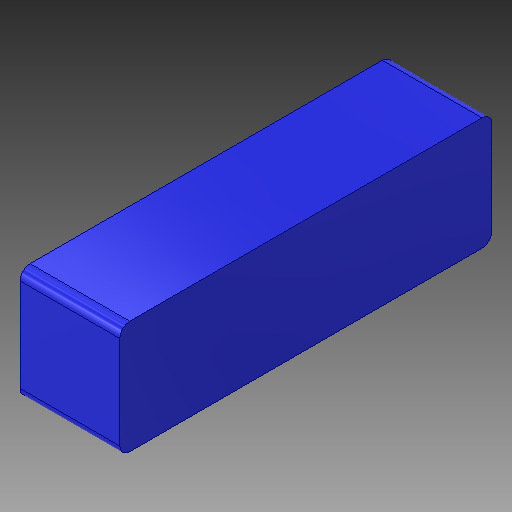
# Autodesk Inventor part: battery
Saved by Autodesk Inventor 2018 (Build 220112000, 112)
## iProperties
Created: 2016-04-08
Part Number: battery
Material: Generic
Document SubType Name: Modeling
Designer: steve
Density: 2.20668 g/cm^3
Appearance: Blue - Wall Paint - Glossy
Mass: 220 g
Surface Area: 147.334 cm^2
Volume: 99.6973 cm^3
Vendor: HobbyKing
Provider: HobbyKing
Author: steve
Autodesk Inventor part; units mm, degrees
ref_plane "YZ Plane" through (0, 0, 0) normal (1, 0, 0) x (0, 1, 0)
ref_plane "XZ Plane" through (0, 0, 0) normal (0, 1, 0) x (-1, 0, 0)
ref_plane "XY Plane" through (0, 0, 0) normal (0, 0, 1) x (1, 0, 0)
sketch "Sketch1" plane through (0, 0, 0) normal (0, 1, 0) x (-1, 0, 0)
  line L0 (-15, 56) -> (15, 56)
  line L1 (15, 56) -> (15, -56)
  line L2 (15, -56) -> (-15, -56)
  line L3 (-15, -56) -> (-15, 56)
  line L4 (-15, 56) -> (15, -56) construction
  line L5 (15, 56) -> (-15, -56) construction
  point P0 (0, 0)
  dimension "d0" = 30
  dimension "d1" = 112
  constraints: 12 end point, 2 midpoint, 2 parallel, 1 horizontal, 1 perpendicular
  measures "d0" distance of L1.end L2.end
  measures "d1" distance of L0.end L1.end
extrude "Extrusion1" add sketch "Sketch1" along normal blind 34
fillet "Fillet1" radius 3 4 edges at (0, 34, -56) (0, 0, -56) (0, 34, 56) (0, 0, 56)
body "Solid1"
